Autodesk Inventor part; units mm, degrees
(part 2 of 5)
  circle A18 centre (0, 0) radius 45 construction
  circle A19 centre (0, 0) radius 45 construction
  line L916 (-38.7494, -0.2217) -> (-38.749, -0.2771)
  line L917 (-38.749, -0.2771) -> (-38.7743, -0.6234)
  line L918 (-38.7743, -0.6234) -> (-38.8288, -0.891)
  line L919 (-38.8288, -0.891) -> (-38.9042, -1.1194)
  line L920 (-38.9042, -1.1194) -> (-38.997, -1.3323)
  line L921 (-38.997, -1.3323) -> (-39.1059, -1.5242)
  line L922 (-39.1059, -1.5242) -> (-39.2291, -1.7067)
  line L923 (-39.2291, -1.7067) -> (-39.366, -1.8725)
  line L924 (-39.366, -1.8725) -> (-39.5158, -2.0289)
  line L925 (-39.5158, -2.0289) -> (-39.6781, -2.1727)
  line L926 (-39.6781, -2.1727) -> (-39.8523, -2.3033)
  line L927 (-39.8523, -2.3033) -> (-40.0379, -2.4272)
  line L928 (-40.0379, -2.4272) -> (-40.2348, -2.5371)
  line L929 (-40.2348, -2.5371) -> (-40.4428, -2.6351)
  line L930 (-40.4428, -2.6351) -> (-40.661, -2.7274)
  line L931 (-41.9049, 3.0266) -> (-42.1825, 3.0578)
  line L932 (-40.661, -2.7274) -> (-40.8898, -2.8078)
  line L933 (-40.8898, -2.8078) -> (-41.1289, -2.8764)
  line L934 (-41.1289, -2.8764) -> (-41.3781, -2.9334)
  line L935 (-41.3781, -2.9334) -> (-41.6367, -2.9845)
  line L936 (-41.9049, -3.0266) -> (-42.1825, -3.0578)
  line L937 (-41.6367, -2.9845) -> (-41.9049, -3.0266)
  line L938 (-40.4428, 2.6351) -> (-40.661, 2.7274)
  line L939 (-42.1825, -3.0578) -> (-42.555, -3.1194)
  line L940 (-42.555, -3.1194) -> (-42.9254, -3.2087)
  line L941 (-43.2942, -3.3167) -> (-43.6617, -3.4402)
  line L942 (-43.6617, -3.4402) -> (-44.0279, -3.5774)
  line L943 (-44.0279, -3.5774) -> (-44.3927, -3.7271)
  line L944 (-42.9254, -3.2087) -> (-43.2942, -3.3167)
  line L945 (-39.5158, 2.0289) -> (-39.6781, 2.1727)
  line L946 (-39.2291, 1.7067) -> (-39.366, 1.8725)
  line L947 (-39.366, 1.8725) -> (-39.5158, 2.0289)
  line L948 (-44.7563, -3.8884) -> (-45.1184, -4.0607)
  line L949 (-47.2601, -5.3011) -> (-47.6113, -5.5395)
  line L950 (-46.9072, -5.0713) -> (-47.2601, -5.3011)
  line L951 (-46.5526, -4.8504) -> (-46.9072, -5.0713)
  line L952 (-46.1963, -4.6386) -> (-46.5526, -4.8504)
  line L953 (-45.8385, -4.4362) -> (-46.1963, -4.6386)
  line L954 (-45.4792, -4.2434) -> (-45.8385, -4.4362)
  line L955 (-45.1184, -4.0607) -> (-45.4792, -4.2434)
  line L956 (-47.6113, -5.5395) -> (-47.9606, -5.7865)
  line L957 (-47.9606, -5.7865) -> (-48.308, -6.0419)
  line L958 (-48.308, -6.0419) -> (-48.6534, -6.3055)
  line L959 (-48.6534, -6.3055) -> (-48.9968, -6.5771)
  line L960 (-48.9968, -6.5771) -> (-49.338, -6.8568)
  line L961 (-49.338, -6.8568) -> (-49.2867, -7.2162)
  line L962 (-49.2867, -7.2162) -> (-49.2328, -7.5752)
  line L963 (-49.2328, -7.5752) -> (-49.1763, -7.9338)
  line L964 (-49.1763, -7.9338) -> (-49.1172, -8.292)
  line L965 (-49.1172, -8.292) -> (-49.0554, -8.6498)
  line L966 (-44.3927, -3.7271) -> (-44.7563, -3.8884)
  line L967 (-39.1059, 1.5242) -> (-39.2291, 1.7067)
  line L968 (-44.3927, 3.7271) -> (-44.7563, 3.8884)
  line L969 (-44.0279, 3.5774) -> (-44.3927, 3.7271)
  line L970 (-43.6617, 3.4402) -> (-44.0279, 3.5774)
  line L971 (-43.2942, 3.3167) -> (-43.6617, 3.4402)
  line L972 (-42.9254, 3.2087) -> (-43.2942, 3.3167)
  line L973 (-42.555, 3.1194) -> (-42.9254, 3.2087)
  line L974 (-44.7563, 3.8884) -> (-45.1184, 4.0607)
  line L975 (-45.1184, 4.0607) -> (-45.4792, 4.2434)
  line L976 (-47.6113, 5.5395) -> (-47.9606, 5.7865)
  line L977 (-47.2601, 5.3011) -> (-47.6113, 5.5395)
  line L978 (-46.9072, 5.0713) -> (-47.2601, 5.3011)
  line L979 (-46.5526, 4.8504) -> (-46.9072, 5.0713)
  line L980 (-46.1963, 4.6386) -> (-46.5526, 4.8504)
  line L981 (-45.8385, 4.4362) -> (-46.1963, 4.6386)
  line L982 (-45.4792, 4.2434) -> (-45.8385, 4.4362)
  line L983 (-47.9606, 5.7865) -> (-48.308, 6.0419)
  line L984 (-48.6534, 6.3055) -> (-48.9968, 6.5771)
  line L985 (-48.9968, 6.5771) -> (-49.338, 6.8568)
  line L986 (-49.338, 6.8568) -> (-49.2867, 7.2162)
  line L987 (-49.2867, 7.2162) -> (-49.2328, 7.5752)
  line L988 (-49.2328, 7.5752) -> (-49.1763, 7.9338)
  line L989 (-49.1763, 7.9338) -> (-49.1172, 8.292)
  line L990 (-49.1172, 8.292) -> (-49.0554, 8.6498)
  line L991 (-48.308, 6.0419) -> (-48.6534, 6.3055)
  line L992 (-38.997, 1.3323) -> (-39.1059, 1.5242)
  line L993 (-38.9042, 1.1194) -> (-38.997, 1.3323)
  line L994 (-38.8288, 0.891) -> (-38.9042, 1.1194)
  line L995 (-38.7743, 0.6234) -> (-38.8288, 0.891)
  line L996 (-38.749, 0.2771) -> (-38.7743, 0.6234)
  line L997 (-38.7494, 0.2217) -> (-38.749, 0.2771)
  line L998 (-38.7496, 0.1663) -> (-38.7494, 0.2217)
  line L999 (-38.7498, 0.1108) -> (-38.7496, 0.1663)
  line L1000 (-38.75, 0.0554) -> (-38.7498, 0.1108)
  line L1001 (-38.75, 0) -> (-38.75, 0.0554)
  line L1002 (-38.0283, -11.529) -> (-38.2367, -11.4659)
  line L1003 (-38.2367, -11.4659) -> (-38.4534, -11.4129)
  line L1004 (-38.4534, -11.4129) -> (-38.6761, -11.377)
  line L1005 (-38.6761, -11.377) -> (-38.905, -11.3561)
  line L1006 (-39.1417, -11.344) -> (-39.3842, -11.3467)
  line L1007 (-39.3842, -11.3467) -> (-39.6323, -11.364)
  line L1008 (-39.6323, -11.364) -> (-39.886, -11.3956)
  line L1009 (-39.886, -11.3956) -> (-40.1465, -11.4361)
  line L1010 (-40.1465, -11.4361) -> (-40.4129, -11.4882)
  line L1011 (-36.4131, -13.2533) -> (-36.3941, -13.3053)
  line L1012 (-36.3941, -13.3053) -> (-36.375, -13.3574)
  line L1013 (-36.375, -13.3574) -> (-36.3559, -13.4094)
  line L1014 (-36.3559, -13.4094) -> (-36.3367, -13.4614)
  line L1015 (-40.6845, -11.5538) -> (-41.0555, -11.6234)
  circle A20 centre (0, 0) radius 45 construction
  circle A21 centre (0, 0) radius 45 construction
  line L1016 (-36.3367, -13.4614) -> (-36.3174, -13.5133)
  line L1017 (-36.3174, -13.5133) -> (-36.2227, -13.8474)
  line L1018 (-36.2227, -13.8474) -> (-36.1824, -14.1175)
  line L1019 (-36.1824, -14.1175) -> (-36.1751, -14.3579)
  line L1020 (-36.1751, -14.3579) -> (-36.1896, -14.5898)
  line L1021 (-36.1896, -14.5898) -> (-36.2262, -14.8073)
  line L1022 (-36.2262, -14.8073) -> (-36.2795, -15.0209)
  line L1023 (-36.2795, -15.0209) -> (-36.3516, -15.2235)
  line L1024 (-36.3516, -15.2235) -> (-36.4388, -15.4218)
  line L1025 (-36.4388, -15.4218) -> (-36.5421, -15.6124)
  line L1026 (-36.5421, -15.6124) -> (-36.6611, -15.7947)
  line L1027 (-36.6611, -15.7947) -> (-36.7931, -15.9746)
  line L1028 (-36.7931, -15.9746) -> (-36.9406, -16.1452)
  line L1029 (-36.9406, -16.1452) -> (-37.1025, -16.3084)
  line L1030 (-37.1025, -16.3084) -> (-37.2761, -16.4698)
  line L1031 (-40.4129, -11.4882) -> (-40.6845, -11.5538)
  line L1032 (-37.2761, -16.4698) -> (-37.4636, -16.6236)
  line L1033 (-37.4636, -16.6236) -> (-37.6648, -16.7698)
  line L1034 (-37.6648, -16.7698) -> (-37.8794, -16.9086)
  line L1035 (-37.8794, -16.9086) -> (-38.105, -17.0451)
  line L1036 (-38.3425, -17.1764) -> (-38.5928, -17.3007)
  line L1037 (-38.105, -17.0451) -> (-38.3425, -17.1764)
  line L1038 (-38.905, -11.3561) -> (-39.1417, -11.344)
  line L1039 (-38.5928, -17.3007) -> (-38.9217, -17.4859)
  line L1040 (-38.9217, -17.4859) -> (-39.2392, -17.6965)
  line L1041 (-39.5489, -17.9241) -> (-39.852, -18.1659)
  line L1042 (-39.852, -18.1659) -> (-40.1491, -18.4201)
  line L1043 (-40.1491, -18.4201) -> (-40.4408, -18.6855)
  line L1044 (-39.2392, -17.6965) -> (-39.5489, -17.9241)
  line L1045 (-37.8267, -11.6087) -> (-38.0283, -11.529)
  line L1046 (-37.447, -11.8133) -> (-37.6324, -11.7044)
  line L1047 (-37.6324, -11.7044) -> (-37.8267, -11.6087)
  line L1048 (-40.7272, -18.9615) -> (-41.0086, -19.2472)
  line L1049 (-42.5969, -21.1453) -> (-42.8453, -21.4895)
  line L1050 (-42.3439, -20.8086) -> (-42.5969, -21.1453)
  line L1051 (-42.0862, -20.4798) -> (-42.3439, -20.8086)
  line L1052 (-41.8239, -20.1589) -> (-42.0862, -20.4798)
  line L1053 (-41.5569, -19.8464) -> (-41.8239, -20.1589)
  line L1054 (-41.2851, -19.5423) -> (-41.5569, -19.8464)
  line L1055 (-41.0086, -19.2472) -> (-41.2851, -19.5423)
  line L1056 (-42.8453, -21.4895) -> (-43.0891, -21.841)
  line L1057 (-43.0891, -21.841) -> (-43.3282, -22.1998)
  line L1058 (-43.3282, -22.1998) -> (-43.5626, -22.5656)
  line L1059 (-43.5626, -22.5656) -> (-43.7924, -22.9383)
  line L1060 (-43.7924, -22.9383) -> (-44.0174, -23.3178)
  line L1061 (-44.0174, -23.3178) -> (-43.8463, -23.638)
  line L1062 (-43.8463, -23.638) -> (-43.6728, -23.957)
  line L1063 (-43.6728, -23.957) -> (-43.4971, -24.2746)
  line L1064 (-43.4971, -24.2746) -> (-43.319, -24.591)
  line L1065 (-43.319, -24.591) -> (-43.1386, -24.9061)
  line L1066 (-40.4408, -18.6855) -> (-40.7272, -18.9615)
  line L1067 (-37.2688, -11.9427) -> (-37.447, -11.8133)
  line L1068 (-42.9903, -11.6809) -> (-43.387, -11.6536)
  line L1069 (-42.5962, -11.6968) -> (-42.9903, -11.6809)
  line L1070 (-42.2052, -11.7005) -> (-42.5962, -11.6968)
  line L1071 (-41.8176, -11.6908) -> (-42.2052, -11.7005)
  line L1072 (-41.4341, -11.6662) -> (-41.8176, -11.6908)
  line L1073 (-41.0555, -11.6234) -> (-41.4341, -11.6662)
  line L1074 (-43.387, -11.6536) -> (-43.7863, -11.6156)
  line L1075 (-43.7863, -11.6156) -> (-44.1878, -11.5673)
  line L1076 (-46.6346, -11.0786) -> (-47.0473, -10.9659)
  line L1077 (-46.223, -11.1825) -> (-46.6346, -11.0786)
  line L1078 (-45.8128, -11.2778) -> (-46.223, -11.1825)
  line L1079 (-45.4041, -11.3641) -> (-45.8128, -11.2778)
  line L1080 (-44.9969, -11.4412) -> (-45.4041, -11.3641)
  line L1081 (-44.5914, -11.509) -> (-44.9969, -11.4412)
  line L1082 (-44.1878, -11.5673) -> (-44.5914, -11.509)
  line L1083 (-47.0473, -10.9659) -> (-47.4611, -10.8448)
  line L1084 (-47.8758, -10.7152) -> (-48.2914, -10.5774)
  line L1085 (-48.2914, -10.5774) -> (-48.7077, -10.4313)
  line L1086 (-48.7077, -10.4313) -> (-48.7824, -10.0761)
  line L1087 (-48.7824, -10.0761) -> (-48.8546, -9.7203)
  line L1088 (-48.8546, -9.7203) -> (-48.9241, -9.3639)
  line L1089 (-48.9241, -9.3639) -> (-48.9911, -9.0071)
  line L1090 (-48.9911, -9.0071) -> (-49.0554, -8.6498)
  line L1091 (-47.4611, -10.8448) -> (-47.8758, -10.7152)
  line L1092 (-37.1009, -12.0858) -> (-37.2688, -11.9427)
  line L1093 (-36.9408, -12.2541) -> (-37.1009, -12.0858)
  line L1094 (-36.7919, -12.4429) -> (-36.9408, -12.2541)
  line L1095 (-36.6492, -12.6758) -> (-36.7919, -12.4429)
  line L1096 (-36.5069, -12.9926) -> (-36.6492, -12.6758)
  line L1097 (-36.4883, -13.0448) -> (-36.5069, -12.9926)
  line L1098 (-36.4696, -13.0969) -> (-36.4883, -13.0448)
  line L1099 (-36.4508, -13.1491) -> (-36.4696, -13.0969)
  line L1100 (-36.432, -13.2012) -> (-36.4508, -13.1491)
  line L1101 (-36.4131, -13.2533) -> (-36.432, -13.2012)
  line L1102 (-31.7918, -23.8401) -> (-32.0092, -23.8521)
  line L1103 (-32.0092, -23.8521) -> (-32.231, -23.8765)
  line L1104 (-32.231, -23.8765) -> (-32.4525, -23.9189)
  line L1105 (-32.4525, -23.9189) -> (-32.6748, -23.9775)
  line L1106 (-32.9013, -24.0471) -> (-33.1282, -24.1326)
  line L1107 (-33.1282, -24.1326) -> (-33.3555, -24.2337)
  line L1108 (-33.3555, -24.2337) -> (-33.583, -24.3502)
  line L1109 (-33.583, -24.3502) -> (-33.814, -24.4773)
  line L1110 (-33.814, -24.4773) -> (-34.0465, -24.6174)
  line L1111 (-29.6842, -24.908) -> (-29.6486, -24.9504)
  line L1112 (-29.6486, -24.9504) -> (-29.6129, -24.9928)
  line L1113 (-29.6129, -24.9928) -> (-29.5771, -25.0351)
  line L1114 (-29.5771, -25.0351) -> (-29.5412, -25.0774)
  line L1115 (-34.2792, -24.772) -> (-34.6041, -24.9642)
  circle A22 centre (0, 0) radius 45 construction
  circle A23 centre (0, 0) radius 45 construction
  line L1116 (-29.5412, -25.0774) -> (-29.5054, -25.1196)
  line L1117 (-29.5054, -25.1196) -> (-29.3021, -25.4012)
  line L1118 (-29.3021, -25.4012) -> (-29.1718, -25.6412)
  line L1119 (-29.1718, -25.6412) -> (-29.0828, -25.8646)
  line L1120 (-29.0828, -25.8646) -> (-29.0171, -26.0875)
  line L1121 (-29.0171, -26.0875) -> (-28.9771, -26.3044)
  line L1122 (-28.9771, -26.3044) -> (-28.9541, -26.5234)
  line L1123 (-28.9541, -26.5234) -> (-28.9525, -26.7384)
  line L1124 (-28.9525, -26.7384) -> (-28.9667, -26.9545)
  line L1125 (-28.9667, -26.9545) -> (-28.9985, -27.169)
  line L1126 (-28.9985, -27.169) -> (-29.0481, -27.381)
  line L1127 (-29.0481, -27.381) -> (-29.1106, -27.5952)
  line L1128 (-29.1106, -27.5952) -> (-29.1908, -27.806)
  line L1129 (-29.1908, -27.806) -> (-29.2872, -28.0147)
  line L1130 (-29.2872, -28.0147) -> (-29.395, -28.2257)
  line L1131 (-34.0465, -24.6174) -> (-34.2792, -24.772)
  line L1132 (-29.395, -28.2257) -> (-29.5186, -28.4343)
  line L1133 (-29.5186, -28.4343) -> (-29.6577, -28.6406)
  line L1134 (-29.6577, -28.6406) -> (-29.8119, -28.8444)
  line L1135 (-29.8119, -28.8444) -> (-29.9772, -29.0498)
  line L1136 (-30.1555, -29.2545) -> (-30.3482, -29.4569)
  line L1137 (-29.9772, -29.0498) -> (-30.1555, -29.2545)
  line L1138 (-32.6748, -23.9775) -> (-32.9013, -24.0471)
  line L1139 (-30.3482, -29.4569) -> (-30.5939, -29.7434)
  line L1140 (-30.5939, -29.7434) -> (-30.8202, -30.0499)
  line L1141 (-31.0334, -30.3697) -> (-31.2355, -30.7005)
  line L1142 (-31.2355, -30.7005) -> (-31.4278, -31.041)
  line L1143 (-31.4278, -31.041) -> (-31.6111, -31.3902)
  line L1144 (-30.8202, -30.0499) -> (-31.0334, -30.3697)
  line L1145 (-31.575, -23.8461) -> (-31.7918, -23.8401)
  line L1146 (-31.1483, -23.9085) -> (-31.3597, -23.8696)
  line L1147 (-31.3597, -23.8696) -> (-31.575, -23.8461)
  line L1148 (-31.7858, -31.7475) -> (-31.9525, -32.1123)
  line L1149 (-32.7959, -34.4391) -> (-32.9116, -34.8475)
  line L1150 (-32.6732, -34.0362) -> (-32.7959, -34.4391)
  line L1151 (-32.5436, -33.639) -> (-32.6732, -34.0362)
  line L1152 (-32.4068, -33.2478) -> (-32.5436, -33.639)
  line L1153 (-32.2628, -32.8628) -> (-32.4068, -33.2478)
  line L1154 (-32.1115, -32.4841) -> (-32.2628, -32.8628)
  line L1155 (-31.9525, -32.1123) -> (-32.1115, -32.4841)
  line L1156 (-32.9116, -34.8475) -> (-33.0204, -35.2612)
  line L1157 (-33.0204, -35.2612) -> (-33.1224, -35.6801)
  line L1158 (-33.1224, -35.6801) -> (-33.2176, -36.1041)
  line L1159 (-33.2176, -36.1041) -> (-33.306, -36.5329)
  line L1160 (-33.306, -36.5329) -> (-33.3877, -36.9664)
  line L1161 (-33.3877, -36.9664) -> (-33.1173, -37.2088)
  line L1162 (-33.1173, -37.2088) -> (-32.8453, -37.4492)
  line L1163 (-32.8453, -37.4492) -> (-32.5715, -37.6876)
  line L1164 (-32.5715, -37.6876) -> (-32.2959, -37.924)
  line L1165 (-32.2959, -37.924) -> (-32.0186, -38.1583)
  line L1166 (-31.6111, -31.3902) -> (-31.7858, -31.7475)
  line L1167 (-30.9366, -23.9692) -> (-31.1483, -23.9085)
  line L1168 (-36.4025, -25.68) -> (-36.7847, -25.7901)
  line L1169 (-36.0268, -25.5601) -> (-36.4025, -25.68)
  line L1170 (-35.6581, -25.4299) -> (-36.0268, -25.5601)
  line L1171 (-35.2972, -25.2883) -> (-35.6581, -25.4299)
  line L1172 (-34.9452, -25.1339) -> (-35.2972, -25.2883)
  line L1173 (-34.6041, -24.9642) -> (-34.9452, -25.1339)
  line L1174 (-36.7847, -25.7901) -> (-37.1729, -25.8909)
  line L1175 (-37.1729, -25.8909) -> (-37.5667, -25.9828)
  line L1176 (-40.0331, -26.3604) -> (-40.4594, -26.3957)
  line L1177 (-39.6108, -26.3174) -> (-40.0331, -26.3604)
  line L1178 (-39.1928, -26.2665) -> (-39.6108, -26.3174)
  line L1179 (-38.7791, -26.2078) -> (-39.1928, -26.2665)
  line L1180 (-38.3701, -26.1411) -> (-38.7791, -26.2078)
  line L1181 (-37.9659, -26.0661) -> (-38.3701, -26.1411)
  line L1182 (-37.5667, -25.9828) -> (-37.9659, -26.0661)
  line L1183 (-40.4594, -26.3957) -> (-40.8897, -26.4234)
  line L1184 (-41.3237, -26.4435) -> (-41.7614, -26.4561)
  line L1185 (-41.7614, -26.4561) -> (-42.2025, -26.4613)
  line L1186 (-42.2025, -26.4613) -> (-42.3943, -26.153)
  line L1187 (-42.3943, -26.153) -> (-42.5838, -25.8433)
  line L1188 (-42.5838, -25.8433) -> (-42.771, -25.5322)
  line L1189 (-42.771, -25.5322) -> (-42.9559, -25.2198)
  line L1190 (-42.9559, -25.2198) -> (-43.1386, -24.9061)
  line L1191 (-40.8897, -26.4234) -> (-41.3237, -26.4435)
  line L1192 (-30.7299, -24.0462) -> (-30.9366, -23.9692)
  line L1193 (-30.5219, -24.1496) -> (-30.7299, -24.0462)
  line L1194 (-30.3173, -24.2761) -> (-30.5219, -24.1496)
  line L1195 (-30.1036, -24.4461) -> (-30.3173, -24.2761)
  line L1196 (-29.8616, -24.6951) -> (-30.1036, -24.4461)
  line L1197 (-29.8262, -24.7378) -> (-29.8616, -24.6951)
  line L1198 (-29.7908, -24.7804) -> (-29.8262, -24.7378)
  line L1199 (-29.7553, -24.823) -> (-29.7908, -24.7804)
  line L1200 (-29.7198, -24.8655) -> (-29.7553, -24.823)
  line L1201 (-29.6842, -24.908) -> (-29.7198, -24.8655)
  line L1202 (-21.7207, -33.2758) -> (-21.9209, -33.3615)
  line L1203 (-21.9209, -33.3615) -> (-22.121, -33.4602)
  line L1204 (-22.121, -33.4602) -> (-22.3146, -33.5758)
  line L1205 (-22.3146, -33.5758) -> (-22.5034, -33.7069)
  line L1206 (-22.6925, -33.8498) -> (-22.8765, -34.0078)
  line L1207 (-22.8765, -34.0078) -> (-23.0555, -34.1805)
  line L1208 (-23.0555, -34.1805) -> (-23.2294, -34.3678)
  line L1209 (-23.2294, -34.3678) -> (-23.403, -34.5662)
  line L1210 (-23.403, -34.5662) -> (-23.5736, -34.7774)
  line L1211 (-19.375, -33.5585) -> (-19.327, -33.5862)
  line L1212 (-19.327, -33.5862) -> (-19.2789, -33.6138)
  line L1213 (-19.2789, -33.6138) -> (-19.2308, -33.6413)
  line L1214 (-19.2308, -33.6413) -> (-19.1827, -33.6688)
  line L1215 (-23.7394, -35.0022) -> (-23.979, -35.294)
  circle A24 centre (0, 0) radius 45 construction
  circle A25 centre (0, 0) radius 45 construction
  line L1216 (-19.1827, -33.6688) -> (-19.1345, -33.6962)
  line L1217 (-19.1345, -33.6962) -> (-18.8473, -33.8913)
  line L1218 (-18.8473, -33.8913) -> (-18.6427, -34.0722)
  line L1219 (-18.6427, -34.0722) -> (-18.4826, -34.2517)
  line L1220 (-18.4826, -34.2517) -> (-18.3447, -34.4386)
  line L1221 (-18.3447, -34.4386) -> (-18.2329, -34.6288)
  line L1222 (-18.2329, -34.6288) -> (-18.1365, -34.8267)
  line L1223 (-18.1365, -34.8267) -> (-18.0614, -35.0282)
  line L1224 (-18.0614, -35.0282) -> (-18.0008, -35.2362)
  line L1225 (-18.0008, -35.2362) -> (-17.9574, -35.4486)
  line L1226 (-17.9574, -35.4486) -> (-17.9314, -35.6648)
  line L1227 (-17.9314, -35.6648) -> (-17.9169, -35.8874)
  line L1228 (-17.9169, -35.8874) -> (-17.9202, -36.1129)
  line L1229 (-17.9202, -36.1129) -> (-17.9393, -36.342)
  line L1230 (-17.9393, -36.342) -> (-17.9685, -36.5772)
  line L1231 (-23.5736, -34.7774) -> (-23.7394, -35.0022)
  line L1232 (-17.9685, -36.5772) -> (-18.0133, -36.8155)
  line L1233 (-18.0133, -36.8155) -> (-18.0734, -37.0569)
  line L1234 (-18.0734, -37.0569) -> (-18.1486, -37.3012)
  line L1235 (-18.1486, -37.3012) -> (-18.2337, -37.5507)
  line L1236 (-18.3313, -37.804) -> (-18.4431, -38.0601)
  line L1237 (-18.2337, -37.5507) -> (-18.3313, -37.804)
  line L1238 (-22.5034, -33.7069) -> (-22.6925, -33.8498)
  line L1239 (-18.4431, -38.0601) -> (-18.576, -38.4134)
  line L1240 (-18.576, -38.4134) -> (-18.6839, -38.7788)
  line L1241 (-18.7748, -39.1522) -> (-18.8516, -39.5322)
  line L1242 (-18.8516, -39.5322) -> (-18.9158, -39.9179)
  line L1243 (-18.9158, -39.9179) -> (-18.9686, -40.3088)
  line L1244 (-18.6839, -38.7788) -> (-18.7748, -39.1522)
  line L1245 (-21.515, -33.2073) -> (-21.7207, -33.2758)
  line L1246 (-21.0926, -33.12) -> (-21.3046, -33.1558)
  line L1247 (-21.3046, -33.1558) -> (-21.515, -33.2073)
  line L1248 (-19.0107, -40.7043) -> (-19.0425, -41.1041)
  line L1249 (-19.0392, -43.579) -> (-19.0083, -44.0023)
  line L1250 (-19.0617, -43.1585) -> (-19.0392, -43.579)
  line L1251 (-19.0757, -42.7409) -> (-19.0617, -43.1585)
  line L1252 (-19.081, -42.3265) -> (-19.0757, -42.7409)
  line L1253 (-19.0774, -41.9154) -> (-19.081, -42.3265)
  line L1254 (-19.0647, -41.5079) -> (-19.0774, -41.9154)
  line L1255 (-19.0425, -41.1041) -> (-19.0647, -41.5079)
  line L1256 (-19.0083, -44.0023) -> (-18.969, -44.4283)
  line L1257 (-18.969, -44.4283) -> (-18.9216, -44.8569)
  line L1258 (-18.9216, -44.8569) -> (-18.866, -45.2878)
  line L1259 (-18.866, -45.2878) -> (-18.8024, -45.721)
  line L1260 (-18.8024, -45.721) -> (-18.7309, -46.1563)
  line L1261 (-18.7309, -46.1563) -> (-18.394, -46.2916)
  line L1262 (-18.394, -46.2916) -> (-18.0561, -46.4245)
  line L1263 (-18.0561, -46.4245) -> (-17.7172, -46.5548)
  line L1264 (-17.7172, -46.5548) -> (-17.3775, -46.6827)
  line L1265 (-17.3775, -46.6827) -> (-17.0368, -46.8081)
  line L1266 (-18.9686, -40.3088) -> (-19.0107, -40.7043)
  line L1267 (-20.8729, -33.1046) -> (-21.0926, -33.12)
  line L1268 (-25.4241, -36.5817) -> (-25.7456, -36.8158)
  line L1269 (-25.1121, -36.3405) -> (-25.4241, -36.5817)
  line L1270 (-24.8101, -36.092) -> (-25.1121, -36.3405)
  line L1271 (-24.5194, -35.8356) -> (-24.8101, -36.092)
  line L1272 (-24.2415, -35.5701) -> (-24.5194, -35.8356)
  line L1273 (-23.979, -35.294) -> (-24.2415, -35.5701)
  line L1274 (-25.7456, -36.8158) -> (-26.0759, -37.0434)
  line L1275 (-26.0759, -37.0434) -> (-26.4145, -37.2644)
  line L1276 (-28.603, -38.4628) -> (-28.9916, -38.6418)
  line L1277 (-28.2209, -38.2779) -> (-28.603, -38.4628)
  line L1278 (-27.8455, -38.0872) -> (-28.2209, -38.2779)
  line L1279 (-27.4768, -37.8905) -> (-27.8455, -38.0872)
  line L1280 (-27.1153, -37.6879) -> (-27.4768, -37.8905)
  line L1281 (-26.7611, -37.4792) -> (-27.1153, -37.6879)
  line L1282 (-26.4145, -37.2644) -> (-26.7611, -37.4792)
  line L1283 (-28.9916, -38.6418) -> (-29.3864, -38.815)
  line L1284 (-29.7874, -38.9823) -> (-30.1943, -39.1439)
  line L1285 (-30.1943, -39.1439) -> (-30.6071, -39.2996)
  line L1286 (-30.6071, -39.2996) -> (-30.8927, -39.0755)
  line L1287 (-30.8927, -39.0755) -> (-31.1767, -38.8493)
  line L1288 (-31.1767, -38.8493) -> (-31.459, -38.621)
  line L1289 (-31.459, -38.621) -> (-31.7397, -38.3907)
  line L1290 (-31.7397, -38.3907) -> (-32.0186, -38.1583)
  line L1291 (-29.3864, -38.815) -> (-29.7874, -38.9823)
  line L1292 (-20.6524, -33.1063) -> (-20.8729, -33.1046)
  line L1293 (-20.4215, -33.1323) -> (-20.6524, -33.1063)
  line L1294 (-20.186, -33.1812) -> (-20.4215, -33.1323)
  line L1295 (-19.9271, -33.2679) -> (-20.186, -33.1812)
  line L1296 (-19.6145, -33.4191) -> (-19.9271, -33.2679)
  line L1297 (-19.5667, -33.4471) -> (-19.6145, -33.4191)
  line L1298 (-19.5188, -33.475) -> (-19.5667, -33.4471)
  line L1299 (-19.4709, -33.5029) -> (-19.5188, -33.475)
  line L1300 (-19.423, -33.5307) -> (-19.4709, -33.5029)
  line L1301 (-19.375, -33.5585) -> (-19.423, -33.5307)
  line L1302 (-9.0298, -38.698) -> (-9.1886, -38.8469)
  line L1303 (-9.1886, -38.8469) -> (-9.3428, -39.0081)
  line L1304 (-9.3428, -39.0081) -> (-9.4853, -39.183)
  line L1305 (-9.4853, -39.183) -> (-9.6179, -39.3708)
  line L1306 (-9.7467, -39.5697) -> (-9.8655, -39.7811)
  line L1307 (-9.8655, -39.7811) -> (-9.9747, -40.0046)
  line L1308 (-9.9747, -40.0046) -> (-10.0741, -40.2401)
  line L1309 (-10.0741, -40.2401) -> (-10.1693, -40.4859)
  line L1310 (-10.1693, -40.4859) -> (-10.2574, -40.7427)
  line L1311 (-6.7289, -38.1613) -> (-6.6743, -38.1709)
  line L1312 (-6.6743, -38.1709) -> (-6.6197, -38.1804)
  line L1313 (-6.6197, -38.1804) -> (-6.5651, -38.1898)
  line L1314 (-6.5651, -38.1898) -> (-6.5105, -38.1992)
  line L1315 (-10.3363, -41.0107) -> (-10.4616, -41.3668)
  circle A26 centre (0, 0) radius 45 construction
  circle A27 centre (0, 0) radius 45 construction
  line L1316 (-6.5105, -38.1992) -> (-6.4558, -38.2084)
  line L1317 (-6.4558, -38.2084) -> (-6.1191, -38.2935)
  line L1318 (-6.1191, -38.2935) -> (-5.8651, -38.3936)
  line L1319 (-5.8651, -38.3936) -> (-5.6532, -38.5075)
  line L1320 (-5.6532, -38.5075) -> (-5.4597, -38.636)
  line L1321 (-5.4597, -38.636) -> (-5.2896, -38.7764)
  line L1322 (-5.2896, -38.7764) -> (-5.1313, -38.9295)
  line L1323 (-5.1313, -38.9295) -> (-4.9918, -39.0931)
  line L1324 (-4.9918, -39.0931) -> (-4.8638, -39.2678)
  line L1325 (-4.8638, -39.2678) -> (-4.7503, -39.4526)
  line L1326 (-4.7503, -39.4526) -> (-4.6519, -39.6468)
  line L1327 (-4.6519, -39.6468) -> (-4.5622, -39.8511)
  line L1328 (-4.5622, -39.8511) -> (-4.4881, -40.0641)
  line L1329 (-4.4881, -40.0641) -> (-4.4278, -40.2859)
  line L1330 (-4.4278, -40.2859) -> (-4.3747, -40.5169)
  line L1331 (-10.2574, -40.7427) -> (-10.3363, -41.0107)
  line L1332 (-4.3747, -40.5169) -> (-4.3353, -40.7562)
  line L1333 (-4.3353, -40.7562) -> (-4.3093, -41.0036)
  line L1334 (-4.3093, -41.0036) -> (-4.2964, -41.2588)
  line L1335 (-4.2964, -41.2588) -> (-4.291, -41.5224)
  line L1336 (-4.2961, -41.7938) -> (-4.3135, -42.0727)
  line L1337 (-4.291, -41.5224) -> (-4.2961, -41.7938)
  line L1338 (-9.6179, -39.3708) -> (-9.7467, -39.5697)
  line L1339 (-4.3135, -42.0727) -> (-4.3176, -42.4502)
  line L1340 (-4.3176, -42.4502) -> (-4.294, -42.8304)
  line L1341 (-4.2517, -43.2124) -> (-4.1939, -43.5958)
  line L1342 (-4.1939, -43.5958) -> (-4.1223, -43.9802)
  line L1343 (-4.1223, -43.9802) -> (-4.0382, -44.3655)
  line L1344 (-4.294, -42.8304) -> (-4.2517, -43.2124)
  line L1345 (-8.8599, -38.5632) -> (-9.0298, -38.698)
  line L1346 (-8.4928, -38.3367) -> (-8.6799, -38.4428)
  line L1347 (-8.6799, -38.4428) -> (-8.8599, -38.5632)
  line L1348 (-3.9425, -44.7515) -> (-3.8357, -45.1381)
  line L1349 (-2.9861, -47.4626) -> (-2.8122, -47.8499)
  line L1350 (-3.1511, -47.0752) -> (-2.9861, -47.4626)
  line L1351 (-3.3071, -46.6876) -> (-3.1511, -47.0752)
  line L1352 (-3.4538, -46.3) -> (-3.3071, -46.6876)
  line L1353 (-3.591, -45.9125) -> (-3.4538, -46.3)
  line L1354 (-3.7184, -45.5251) -> (-3.591, -45.9125)
  line L1355 (-3.8357, -45.1381) -> (-3.7184, -45.5251)
  line L1356 (-2.8122, -47.8499) -> (-2.6297, -48.2368)
  line L1357 (-2.6297, -48.2368) -> (-2.4385, -48.6232)
  line L1358 (-2.4385, -48.6232) -> (-2.2389, -49.0092)
  line L1359 (-2.2389, -49.0092) -> (-2.031, -49.3945)
  line L1360 (-2.031, -49.3945) -> (-1.8149, -49.7791)
  line L1361 (-1.8149, -49.7791) -> (-1.452, -49.791)
  line L1362 (-1.452, -49.791) -> (-1.0891, -49.8003)
  line L1363 (-1.0891, -49.8003) -> (-0.7261, -49.8069)
  line L1364 (-0.7261, -49.8069) -> (-0.363, -49.8108)
  line L1365 (-0.363, -49.8108) -> (0, -49.8122)
  line L1366 (-4.0382, -44.3655) -> (-3.9425, -44.7515)
  line L1367 (-8.2917, -38.2471) -> (-8.4928, -38.3367)
  line L1368 (-11.3792, -43.0711) -> (-11.6012, -43.4011)
  line L1369 (-11.1684, -42.7378) -> (-11.3792, -43.0711)
  line L1370 (-10.9697, -42.401) -> (-11.1684, -42.7378)
  line L1371 (-10.7842, -42.0605) -> (-10.9697, -42.401)
  line L1372 (-10.6138, -41.716) -> (-10.7842, -42.0605)
  line L1373 (-10.4616, -41.3668) -> (-10.6138, -41.716)
  line L1374 (-11.6012, -43.4011) -> (-11.8338, -43.7278)
  line L1375 (-11.8338, -43.7278) -> (-12.0764, -44.0514)
  line L1376 (-13.723, -45.926) -> (-14.0269, -46.2271)
  line L1377 (-13.4272, -45.6216) -> (-13.723, -45.926)
  line L1378 (-13.1396, -45.314) -> (-13.4272, -45.6216)
  line L1379 (-12.8605, -45.0031) -> (-13.1396, -45.314)
  line L1380 (-12.59, -44.689) -> (-12.8605, -45.0031)
  line L1381 (-12.3286, -44.3718) -> (-12.59, -44.689)
  line L1382 (-12.0764, -44.0514) -> (-12.3286, -44.3718)
  line L1383 (-14.0269, -46.2271) -> (-14.3387, -46.5249)
  line L1384 (-14.6582, -46.8193) -> (-14.9854, -47.1103)
  line L1385 (-14.9854, -47.1103) -> (-15.32, -47.3978)
  line L1386 (-15.32, -47.3978) -> (-15.6651, -47.2849)
  line L1387 (-15.6651, -47.2849) -> (-16.0093, -47.1694)
  line L1388 (-16.0093, -47.1694) -> (-16.3527, -47.0515)
  line L1389 (-16.3527, -47.0515) -> (-16.6952, -46.9311)
  line L1390 (-16.6952, -46.9311) -> (-17.0368, -46.8081)
  line L1391 (-14.3387, -46.5249) -> (-14.6582, -46.8193)
  line L1392 (-8.0839, -38.1732) -> (-8.2917, -38.2471)
  line L1393 (-7.8581, -38.1187) -> (-8.0839, -38.1732)
  line L1394 (-7.62, -38.0842) -> (-7.8581, -38.1187)
  line L1395 (-7.347, -38.077) -> (-7.62, -38.0842)
  line L1396 (-7.0016, -38.1122) -> (-7.347, -38.077)
  line L1397 (-6.9471, -38.1222) -> (-7.0016, -38.1122)
  line L1398 (-6.8925, -38.1321) -> (-6.9471, -38.1222)
  line L1399 (-6.838, -38.1419) -> (-6.8925, -38.1321)
  line L1400 (-6.7834, -38.1516) -> (-6.838, -38.1419)
  line L1401 (-6.7289, -38.1613) -> (-6.7834, -38.1516)
  line L1402 (4.7503, -39.4526) -> (4.6519, -39.6468)
  line L1403 (4.6519, -39.6468) -> (4.5622, -39.8511)
  line L1404 (4.5622, -39.8511) -> (4.4881, -40.0641)
  line L1405 (4.4881, -40.0641) -> (4.4278, -40.2859)
  line L1406 (4.3747, -40.5169) -> (4.3353, -40.7562)
  line L1407 (4.3353, -40.7562) -> (4.3093, -41.0036)
  line L1408 (4.3093, -41.0036) -> (4.2964, -41.2588)
  line L1409 (4.2964, -41.2588) -> (4.291, -41.5224)
  line L1410 (4.291, -41.5224) -> (4.2961, -41.7938)
  line L1411 (6.7289, -38.1613) -> (6.7834, -38.1516)
  line L1412 (6.7834, -38.1516) -> (6.838, -38.1419)
  line L1413 (6.838, -38.1419) -> (6.8925, -38.1321)
  line L1414 (6.8925, -38.1321) -> (6.9471, -38.1222)
  line L1415 (4.3135, -42.0727) -> (4.3176, -42.4502)
  circle A28 centre (0, 0) radius 45 construction
  circle A29 centre (0, 0) radius 45 construction
  line L1416 (6.9471, -38.1222) -> (7.0016, -38.1122)
  line L1417 (7.0016, -38.1122) -> (7.347, -38.077)
  line L1418 (7.347, -38.077) -> (7.62, -38.0842)
  line L1419 (7.62, -38.0842) -> (7.8581, -38.1187)
  line L1420 (7.8581, -38.1187) -> (8.0839, -38.1732)
  line L1421 (8.0839, -38.1732) -> (8.2917, -38.2471)
  line L1422 (8.2917, -38.2471) -> (8.4928, -38.3367)
  line L1423 (8.4928, -38.3367) -> (8.6799, -38.4428)
  line L1424 (8.6799, -38.4428) -> (8.8599, -38.5632)
  line L1425 (8.8599, -38.5632) -> (9.0298, -38.698)
  line L1426 (9.0298, -38.698) -> (9.1886, -38.8469)
  line L1427 (9.1886, -38.8469) -> (9.3428, -39.0081)
  line L1428 (9.3428, -39.0081) -> (9.4853, -39.183)
  line L1429 (9.4853, -39.183) -> (9.6179, -39.3708)
  line L1430 (9.6179, -39.3708) -> (9.7467, -39.5697)
  line L1431 (4.2961, -41.7938) -> (4.3135, -42.0727)
  line L1432 (9.7467, -39.5697) -> (9.8655, -39.7811)
  line L1433 (9.8655, -39.7811) -> (9.9747, -40.0046)
  line L1434 (9.9747, -40.0046) -> (10.0741, -40.2401)
  line L1435 (10.0741, -40.2401) -> (10.1693, -40.4859)
  line L1436 (10.2574, -40.7427) -> (10.3363, -41.0107)
  line L1437 (10.1693, -40.4859) -> (10.2574, -40.7427)
  line L1438 (4.4278, -40.2859) -> (4.3747, -40.5169)
  line L1439 (10.3363, -41.0107) -> (10.4616, -41.3668)
  line L1440 (10.4616, -41.3668) -> (10.6138, -41.716)
  line L1441 (10.7842, -42.0605) -> (10.9697, -42.401)
  line L1442 (10.9697, -42.401) -> (11.1684, -42.7378)
  line L1443 (11.1684, -42.7378) -> (11.3792, -43.0711)
  line L1444 (10.6138, -41.716) -> (10.7842, -42.0605)
  line L1445 (4.8638, -39.2678) -> (4.7503, -39.4526)
  line L1446 (5.1313, -38.9295) -> (4.9918, -39.0931)
  line L1447 (4.9918, -39.0931) -> (4.8638, -39.2678)
  line L1448 (11.6012, -43.4011) -> (11.8338, -43.7278)
  line L1449 (13.4272, -45.6216) -> (13.723, -45.926)
  line L1450 (13.1396, -45.314) -> (13.4272, -45.6216)
  line L1451 (12.8605, -45.0031) -> (13.1396, -45.314)
  line L1452 (12.59, -44.689) -> (12.8605, -45.0031)
  line L1453 (12.3286, -44.3718) -> (12.59, -44.689)
  line L1454 (12.0764, -44.0514) -> (12.3286, -44.3718)
  line L1455 (11.8338, -43.7278) -> (12.0764, -44.0514)
  line L1456 (13.723, -45.926) -> (14.0269, -46.2271)
  line L1457 (14.0269, -46.2271) -> (14.3387, -46.5249)
  line L1458 (14.3387, -46.5249) -> (14.6582, -46.8193)
  line L1459 (14.6582, -46.8193) -> (14.9854, -47.1103)
  line L1460 (14.9854, -47.1103) -> (15.32, -47.3978)
  line L1461 (15.32, -47.3978) -> (15.6651, -47.2849)
  line L1462 (15.6651, -47.2849) -> (16.0093, -47.1694)
  line L1463 (16.0093, -47.1694) -> (16.3527, -47.0515)
  line L1464 (16.3527, -47.0515) -> (16.6952, -46.9311)
  line L1465 (16.6952, -46.9311) -> (17.0368, -46.8081)
  line L1466 (11.3792, -43.0711) -> (11.6012, -43.4011)
  line L1467 (5.2896, -38.7764) -> (5.1313, -38.9295)
  line L1468 (4.0382, -44.3655) -> (3.9425, -44.7515)
  line L1469 (4.1223, -43.9802) -> (4.0382, -44.3655)
  line L1470 (4.1939, -43.5958) -> (4.1223, -43.9802)
  line L1471 (4.2517, -43.2124) -> (4.1939, -43.5958)
  line L1472 (4.294, -42.8304) -> (4.2517, -43.2124)
  line L1473 (4.3176, -42.4502) -> (4.294, -42.8304)
  line L1474 (3.9425, -44.7515) -> (3.8357, -45.1381)
  line L1475 (3.8357, -45.1381) -> (3.7184, -45.5251)
  line L1476 (2.8122, -47.8499) -> (2.6297, -48.2368)
  line L1477 (2.9861, -47.4626) -> (2.8122, -47.8499)
  line L1478 (3.1511, -47.0752) -> (2.9861, -47.4626)
  line L1479 (3.3071, -46.6876) -> (3.1511, -47.0752)
  line L1480 (3.4538, -46.3) -> (3.3071, -46.6876)
  line L1481 (3.591, -45.9125) -> (3.4538, -46.3)
  line L1482 (3.7184, -45.5251) -> (3.591, -45.9125)
  line L1483 (2.6297, -48.2368) -> (2.4385, -48.6232)
  line L1484 (2.2389, -49.0092) -> (2.031, -49.3945)
  line L1485 (2.031, -49.3945) -> (1.8149, -49.7791)
  line L1486 (1.8149, -49.7791) -> (1.452, -49.791)
  line L1487 (1.452, -49.791) -> (1.0891, -49.8003)
  line L1488 (1.0891, -49.8003) -> (0.7261, -49.8069)
  line L1489 (0.7261, -49.8069) -> (0.363, -49.8108)
  line L1490 (0.363, -49.8108) -> (0, -49.8122)
  line L1491 (2.4385, -48.6232) -> (2.2389, -49.0092)
  line L1492 (5.4597, -38.636) -> (5.2896, -38.7764)
  line L1493 (5.6532, -38.5075) -> (5.4597, -38.636)
  line L1494 (5.8651, -38.3936) -> (5.6532, -38.5075)
  line L1495 (6.1191, -38.2935) -> (5.8651, -38.3936)
  line L1496 (6.4558, -38.2084) -> (6.1191, -38.2935)
  line L1497 (6.5105, -38.1992) -> (6.4558, -38.2084)
  line L1498 (6.5651, -38.1898) -> (6.5105, -38.1992)
  line L1499 (6.6197, -38.1804) -> (6.5651, -38.1898)
  line L1500 (6.6743, -38.1709) -> (6.6197, -38.1804)
  line L1501 (6.7289, -38.1613) -> (6.6743, -38.1709)
  line L1502 (17.9574, -35.4486) -> (17.9314, -35.6648)
  line L1503 (17.9314, -35.6648) -> (17.9169, -35.8874)
  line L1504 (17.9169, -35.8874) -> (17.9202, -36.1129)
  line L1505 (17.9202, -36.1129) -> (17.9393, -36.342)
  line L1506 (17.9685, -36.5772) -> (18.0133, -36.8155)
  line L1507 (18.0133, -36.8155) -> (18.0734, -37.0569)
  line L1508 (18.0734, -37.0569) -> (18.1486, -37.3012)
  line L1509 (18.1486, -37.3012) -> (18.2337, -37.5507)
  line L1510 (18.2337, -37.5507) -> (18.3313, -37.804)
  line L1511 (19.375, -33.5585) -> (19.423, -33.5307)
  line L1512 (19.423, -33.5307) -> (19.4709, -33.5029)
  line L1513 (19.4709, -33.5029) -> (19.5188, -33.475)
  line L1514 (19.5188, -33.475) -> (19.5667, -33.4471)
  line L1515 (18.4431, -38.0601) -> (18.576, -38.4134)
  circle A30 centre (0, 0) radius 45 construction
  circle A31 centre (0, 0) radius 45 construction
  line L1516 (19.5667, -33.4471) -> (19.6145, -33.4191)
  line L1517 (19.6145, -33.4191) -> (19.9271, -33.2679)
  line L1518 (19.9271, -33.2679) -> (20.186, -33.1812)
  line L1519 (20.186, -33.1812) -> (20.4215, -33.1323)
  line L1520 (20.4215, -33.1323) -> (20.6524, -33.1063)
  line L1521 (20.6524, -33.1063) -> (20.8729, -33.1046)
  line L1522 (20.8729, -33.1046) -> (21.0926, -33.12)
  line L1523 (21.0926, -33.12) -> (21.3046, -33.1558)
  line L1524 (21.3046, -33.1558) -> (21.515, -33.2073)
  line L1525 (21.515, -33.2073) -> (21.7207, -33.2758)
  line L1526 (21.7207, -33.2758) -> (21.9209, -33.3615)
  line L1527 (21.9209, -33.3615) -> (22.121, -33.4602)
  line L1528 (22.121, -33.4602) -> (22.3146, -33.5758)
  line L1529 (22.3146, -33.5758) -> (22.5034, -33.7069)
  line L1530 (22.5034, -33.7069) -> (22.6925, -33.8498)
  line L1531 (18.3313, -37.804) -> (18.4431, -38.0601)
  line L1532 (22.6925, -33.8498) -> (22.8765, -34.0078)
  line L1533 (22.8765, -34.0078) -> (23.0555, -34.1805)
  line L1534 (23.0555, -34.1805) -> (23.2294, -34.3678)
  line L1535 (23.2294, -34.3678) -> (23.403, -34.5662)
  line L1536 (23.5736, -34.7774) -> (23.7394, -35.0022)
  line L1537 (23.403, -34.5662) -> (23.5736, -34.7774)
  line L1538 (17.9393, -36.342) -> (17.9685, -36.5772)
  line L1539 (23.7394, -35.0022) -> (23.979, -35.294)
  line L1540 (23.979, -35.294) -> (24.2415, -35.5701)
  line L1541 (24.5194, -35.8356) -> (24.8101, -36.092)
  line L1542 (24.8101, -36.092) -> (25.1121, -36.3405)
  line L1543 (25.1121, -36.3405) -> (25.4241, -36.5817)
  line L1544 (24.2415, -35.5701) -> (24.5194, -35.8356)
  line L1545 (18.0008, -35.2362) -> (17.9574, -35.4486)
  line L1546 (18.1365, -34.8267) -> (18.0614, -35.0282)
  line L1547 (18.0614, -35.0282) -> (18.0008, -35.2362)
  line L1548 (25.7456, -36.8158) -> (26.0759, -37.0434)
  line L1549 (28.2209, -38.2779) -> (28.603, -38.4628)
  line L1550 (27.8455, -38.0872) -> (28.2209, -38.2779)
  line L1551 (27.4768, -37.8905) -> (27.8455, -38.0872)
  line L1552 (27.1153, -37.6879) -> (27.4768, -37.8905)
  line L1553 (26.7611, -37.4792) -> (27.1153, -37.6879)
  line L1554 (26.4145, -37.2644) -> (26.7611, -37.4792)
  line L1555 (26.0759, -37.0434) -> (26.4145, -37.2644)
  line L1556 (28.603, -38.4628) -> (28.9916, -38.6418)
  line L1557 (28.9916, -38.6418) -> (29.3864, -38.815)
  line L1558 (29.3864, -38.815) -> (29.7874, -38.9823)
  line L1559 (29.7874, -38.9823) -> (30.1943, -39.1439)
  line L1560 (30.1943, -39.1439) -> (30.6071, -39.2996)
  line L1561 (30.6071, -39.2996) -> (30.8927, -39.0755)
  line L1562 (30.8927, -39.0755) -> (31.1767, -38.8493)
  line L1563 (31.1767, -38.8493) -> (31.459, -38.621)
  line L1564 (31.459, -38.621) -> (31.7397, -38.3907)
  line L1565 (31.7397, -38.3907) -> (32.0186, -38.1583)
  line L1566 (25.4241, -36.5817) -> (25.7456, -36.8158)
  line L1567 (18.2329, -34.6288) -> (18.1365, -34.8267)
  line L1568 (18.9686, -40.3088) -> (19.0107, -40.7043)
  line L1569 (18.9158, -39.9179) -> (18.9686, -40.3088)
  line L1570 (18.8516, -39.5322) -> (18.9158, -39.9179)
  line L1571 (18.7748, -39.1522) -> (18.8516, -39.5322)
  line L1572 (18.6839, -38.7788) -> (18.7748, -39.1522)
  line L1573 (18.576, -38.4134) -> (18.6839, -38.7788)
  line L1574 (19.0107, -40.7043) -> (19.0425, -41.1041)
  line L1575 (19.0425, -41.1041) -> (19.0647, -41.5079)
  line L1576 (19.0083, -44.0023) -> (18.969, -44.4283)
  line L1577 (19.0392, -43.579) -> (19.0083, -44.0023)
  line L1578 (19.0617, -43.1585) -> (19.0392, -43.579)
  line L1579 (19.0757, -42.7409) -> (19.0617, -43.1585)
  line L1580 (19.081, -42.3265) -> (19.0757, -42.7409)
  line L1581 (19.0774, -41.9154) -> (19.081, -42.3265)
  line L1582 (19.0647, -41.5079) -> (19.0774, -41.9154)
  line L1583 (18.969, -44.4283) -> (18.9216, -44.8569)
  line L1584 (18.866, -45.2878) -> (18.8024, -45.721)
  line L1585 (18.8024, -45.721) -> (18.7309, -46.1563)
  line L1586 (18.7309, -46.1563) -> (18.394, -46.2916)
  line L1587 (18.394, -46.2916) -> (18.0561, -46.4245)
  line L1588 (18.0561, -46.4245) -> (17.7172, -46.5548)
  line L1589 (17.7172, -46.5548) -> (17.3775, -46.6827)
  line L1590 (17.3775, -46.6827) -> (17.0368, -46.8081)
  line L1591 (18.9216, -44.8569) -> (18.866, -45.2878)
  line L1592 (18.3447, -34.4386) -> (18.2329, -34.6288)
  line L1593 (18.4826, -34.2517) -> (18.3447, -34.4386)
  line L1594 (18.6427, -34.0722) -> (18.4826, -34.2517)
  line L1595 (18.8473, -33.8913) -> (18.6427, -34.0722)
  line L1596 (19.1345, -33.6962) -> (18.8473, -33.8913)
  line L1597 (19.1827, -33.6688) -> (19.1345, -33.6962)
  line L1598 (19.2308, -33.6413) -> (19.1827, -33.6688)
  line L1599 (19.2789, -33.6138) -> (19.2308, -33.6413)
  line L1600 (19.327, -33.5862) -> (19.2789, -33.6138)
  line L1601 (19.375, -33.5585) -> (19.327, -33.5862)
  line L1602 (28.9985, -27.169) -> (29.0481, -27.381)
  line L1603 (29.0481, -27.381) -> (29.1106, -27.5952)
  line L1604 (29.1106, -27.5952) -> (29.1908, -27.806)
  line L1605 (29.1908, -27.806) -> (29.2872, -28.0147)
  line L1606 (29.395, -28.2257) -> (29.5186, -28.4343)
  line L1607 (29.5186, -28.4343) -> (29.6577, -28.6406)
  line L1608 (29.6577, -28.6406) -> (29.8119, -28.8444)
  line L1609 (29.8119, -28.8444) -> (29.9772, -29.0498)
  line L1610 (29.9772, -29.0498) -> (30.1555, -29.2545)
  line L1611 (29.6842, -24.908) -> (29.7198, -24.8655)
  line L1612 (29.7198, -24.8655) -> (29.7553, -24.823)
  line L1613 (29.7553, -24.823) -> (29.7908, -24.7804)
  line L1614 (29.7908, -24.7804) -> (29.8262, -24.7378)
  line L1615 (30.3482, -29.4569) -> (30.5939, -29.7434)
  circle A32 centre (0, 0) radius 45 construction
  circle A33 centre (0, 0) radius 45 construction
  line L1616 (29.8262, -24.7378) -> (29.8616, -24.6951)
  line L1617 (29.8616, -24.6951) -> (30.1036, -24.4461)
  line L1618 (30.1036, -24.4461) -> (30.3173, -24.2761)
  line L1619 (30.3173, -24.2761) -> (30.5219, -24.1496)
  line L1620 (30.5219, -24.1496) -> (30.7299, -24.0462)
  line L1621 (30.7299, -24.0462) -> (30.9366, -23.9692)
  line L1622 (30.9366, -23.9692) -> (31.1483, -23.9085)
  line L1623 (31.1483, -23.9085) -> (31.3597, -23.8696)
  line L1624 (31.3597, -23.8696) -> (31.575, -23.8461)
  line L1625 (31.575, -23.8461) -> (31.7918, -23.8401)
  line L1626 (31.7918, -23.8401) -> (32.0092, -23.8521)
  line L1627 (32.0092, -23.8521) -> (32.231, -23.8765)
  line L1628 (32.231, -23.8765) -> (32.4525, -23.9189)
  line L1629 (32.4525, -23.9189) -> (32.6748, -23.9775)
  line L1630 (32.6748, -23.9775) -> (32.9013, -24.0471)
  line L1631 (30.1555, -29.2545) -> (30.3482, -29.4569)
  line L1632 (32.9013, -24.0471) -> (33.1282, -24.1326)
  line L1633 (33.1282, -24.1326) -> (33.3555, -24.2337)
  line L1634 (33.3555, -24.2337) -> (33.583, -24.3502)
  line L1635 (33.583, -24.3502) -> (33.814, -24.4773)
  line L1636 (34.0465, -24.6174) -> (34.2792, -24.772)
  line L1637 (33.814, -24.4773) -> (34.0465, -24.6174)
  line L1638 (29.2872, -28.0147) -> (29.395, -28.2257)
  line L1639 (34.2792, -24.772) -> (34.6041, -24.9642)
  line L1640 (34.6041, -24.9642) -> (34.9452, -25.1339)
  line L1641 (35.2972, -25.2883) -> (35.6581, -25.4299)
  line L1642 (35.6581, -25.4299) -> (36.0268, -25.5601)
  line L1643 (36.0268, -25.5601) -> (36.4025, -25.68)
  line L1644 (34.9452, -25.1339) -> (35.2972, -25.2883)
  line L1645 (28.9667, -26.9545) -> (28.9985, -27.169)
  line L1646 (28.9541, -26.5234) -> (28.9525, -26.7384)
  line L1647 (28.9525, -26.7384) -> (28.9667, -26.9545)
  line L1648 (36.7847, -25.7901) -> (37.1729, -25.8909)
  line L1649 (39.6108, -26.3174) -> (40.0331, -26.3604)
  line L1650 (39.1928, -26.2665) -> (39.6108, -26.3174)
  line L1651 (38.7791, -26.2078) -> (39.1928, -26.2665)
  line L1652 (38.3701, -26.1411) -> (38.7791, -26.2078)
  line L1653 (37.9659, -26.0661) -> (38.3701, -26.1411)
  line L1654 (37.5667, -25.9828) -> (37.9659, -26.0661)
  line L1655 (37.1729, -25.8909) -> (37.5667, -25.9828)
  line L1656 (40.0331, -26.3604) -> (40.4594, -26.3957)
  line L1657 (40.4594, -26.3957) -> (40.8897, -26.4234)
  line L1658 (40.8897, -26.4234) -> (41.3237, -26.4435)
  line L1659 (41.3237, -26.4435) -> (41.7614, -26.4561)
  line L1660 (41.7614, -26.4561) -> (42.2025, -26.4613)
  line L1661 (42.2025, -26.4613) -> (42.3943, -26.153)
  line L1662 (42.3943, -26.153) -> (42.5838, -25.8433)
  line L1663 (42.5838, -25.8433) -> (42.771, -25.5322)
  line L1664 (42.771, -25.5322) -> (42.9559, -25.2198)
  line L1665 (42.9559, -25.2198) -> (43.1386, -24.9061)
  line L1666 (36.4025, -25.68) -> (36.7847, -25.7901)
  line L1667 (28.9771, -26.3044) -> (28.9541, -26.5234)
  line L1668 (31.6111, -31.3902) -> (31.7858, -31.7475)
  line L1669 (31.4278, -31.041) -> (31.6111, -31.3902)
  line L1670 (31.2355, -30.7005) -> (31.4278, -31.041)
  line L1671 (31.0334, -30.3697) -> (31.2355, -30.7005)
  line L1672 (30.8202, -30.0499) -> (31.0334, -30.3697)
  line L1673 (30.5939, -29.7434) -> (30.8202, -30.0499)
  line L1674 (31.7858, -31.7475) -> (31.9525, -32.1123)
  line L1675 (31.9525, -32.1123) -> (32.1115, -32.4841)
  line L1676 (32.9116, -34.8475) -> (33.0204, -35.2612)
  line L1677 (32.7959, -34.4391) -> (32.9116, -34.8475)
  line L1678 (32.6732, -34.0362) -> (32.7959, -34.4391)
  line L1679 (32.5436, -33.639) -> (32.6732, -34.0362)
  line L1680 (32.4068, -33.2478) -> (32.5436, -33.639)
  line L1681 (32.2628, -32.8628) -> (32.4068, -33.2478)
  line L1682 (32.1115, -32.4841) -> (32.2628, -32.8628)
  line L1683 (33.0204, -35.2612) -> (33.1224, -35.6801)
  line L1684 (33.2176, -36.1041) -> (33.306, -36.5329)
  line L1685 (33.306, -36.5329) -> (33.3877, -36.9664)
  line L1686 (33.3877, -36.9664) -> (33.1173, -37.2088)
  line L1687 (33.1173, -37.2088) -> (32.8453, -37.4492)
  line L1688 (32.8453, -37.4492) -> (32.5715, -37.6876)
  line L1689 (32.5715, -37.6876) -> (32.2959, -37.924)
  line L1690 (32.2959, -37.924) -> (32.0186, -38.1583)
  line L1691 (33.1224, -35.6801) -> (33.2176, -36.1041)
  line L1692 (29.0171, -26.0875) -> (28.9771, -26.3044)
  line L1693 (29.0828, -25.8646) -> (29.0171, -26.0875)
  line L1694 (29.1718, -25.6412) -> (29.0828, -25.8646)
  line L1695 (29.3021, -25.4012) -> (29.1718, -25.6412)
  line L1696 (29.5054, -25.1196) -> (29.3021, -25.4012)
  line L1697 (29.5412, -25.0774) -> (29.5054, -25.1196)
  line L1698 (29.5771, -25.0351) -> (29.5412, -25.0774)
  line L1699 (29.6129, -24.9928) -> (29.5771, -25.0351)
  line L1700 (29.6486, -24.9504) -> (29.6129, -24.9928)
  line L1701 (29.6842, -24.908) -> (29.6486, -24.9504)
  line L1702 (36.5421, -15.6124) -> (36.6611, -15.7947)
  line L1703 (36.6611, -15.7947) -> (36.7931, -15.9746)
  line L1704 (36.7931, -15.9746) -> (36.9406, -16.1452)
  line L1705 (36.9406, -16.1452) -> (37.1025, -16.3084)
  line L1706 (37.2761, -16.4698) -> (37.4636, -16.6236)
  line L1707 (37.4636, -16.6236) -> (37.6648, -16.7698)
  line L1708 (37.6648, -16.7698) -> (37.8794, -16.9086)
  line L1709 (37.8794, -16.9086) -> (38.105, -17.0451)
  line L1710 (38.105, -17.0451) -> (38.3425, -17.1764)
  line L1711 (36.4131, -13.2533) -> (36.432, -13.2012)
  line L1712 (36.432, -13.2012) -> (36.4508, -13.1491)
  line L1713 (36.4508, -13.1491) -> (36.4696, -13.0969)
  line L1714 (36.4696, -13.0969) -> (36.4883, -13.0448)
  line L1715 (38.5928, -17.3007) -> (38.9217, -17.4859)
  circle A34 centre (0, 0) radius 45 construction
  circle A35 centre (0, 0) radius 45 construction
  line L1716 (36.4883, -13.0448) -> (36.5069, -12.9926)
  line L1717 (36.5069, -12.9926) -> (36.6492, -12.6758)
  line L1718 (36.6492, -12.6758) -> (36.7919, -12.4429)
  line L1719 (36.7919, -12.4429) -> (36.9408, -12.2541)
  line L1720 (36.9408, -12.2541) -> (37.1009, -12.0858)
  line L1721 (37.1009, -12.0858) -> (37.2688, -11.9427)
  line L1722 (37.2688, -11.9427) -> (37.447, -11.8133)
  line L1723 (37.447, -11.8133) -> (37.6324, -11.7044)
  line L1724 (37.6324, -11.7044) -> (37.8267, -11.6087)
  line L1725 (37.8267, -11.6087) -> (38.0283, -11.529)
  line L1726 (38.0283, -11.529) -> (38.2367, -11.4659)
  line L1727 (38.2367, -11.4659) -> (38.4534, -11.4129)
  line L1728 (38.4534, -11.4129) -> (38.6761, -11.377)
  line L1729 (38.6761, -11.377) -> (38.905, -11.3561)
  line L1730 (38.905, -11.3561) -> (39.1417, -11.344)
  line L1731 (38.3425, -17.1764) -> (38.5928, -17.3007)
  line L1732 (39.1417, -11.344) -> (39.3842, -11.3467)
  line L1733 (39.3842, -11.3467) -> (39.6323, -11.364)
  line L1734 (39.6323, -11.364) -> (39.886, -11.3956)
  line L1735 (39.886, -11.3956) -> (40.1465, -11.4361)
  line L1736 (40.4129, -11.4882) -> (40.6845, -11.5538)
  line L1737 (40.1465, -11.4361) -> (40.4129, -11.4882)
  line L1738 (37.1025, -16.3084) -> (37.2761, -16.4698)
  line L1739 (40.6845, -11.5538) -> (41.0555, -11.6234)
  line L1740 (41.0555, -11.6234) -> (41.4341, -11.6662)
  line L1741 (41.8176, -11.6908) -> (42.2052, -11.7005)
  line L1742 (42.2052, -11.7005) -> (42.5962, -11.6968)
  line L1743 (42.5962, -11.6968) -> (42.9903, -11.6809)
  line L1744 (41.4341, -11.6662) -> (41.8176, -11.6908)
  line L1745 (36.4388, -15.4218) -> (36.5421, -15.6124)
  line L1746 (36.2795, -15.0209) -> (36.3516, -15.2235)
  line L1747 (36.3516, -15.2235) -> (36.4388, -15.4218)
  line L1748 (43.387, -11.6536) -> (43.7863, -11.6156)
  line L1749 (46.223, -11.1825) -> (46.6346, -11.0786)
  line L1750 (45.8128, -11.2778) -> (46.223, -11.1825)
  line L1751 (45.4041, -11.3641) -> (45.8128, -11.2778)
  line L1752 (44.9969, -11.4412) -> (45.4041, -11.3641)
  line L1753 (44.5914, -11.509) -> (44.9969, -11.4412)
  line L1754 (44.1878, -11.5673) -> (44.5914, -11.509)
  line L1755 (43.7863, -11.6156) -> (44.1878, -11.5673)
  line L1756 (46.6346, -11.0786) -> (47.0473, -10.9659)
  line L1757 (47.0473, -10.9659) -> (47.4611, -10.8448)
  line L1758 (47.4611, -10.8448) -> (47.8758, -10.7152)
  line L1759 (47.8758, -10.7152) -> (48.2914, -10.5774)
  line L1760 (48.2914, -10.5774) -> (48.7077, -10.4313)
  line L1761 (48.7077, -10.4313) -> (48.7824, -10.0761)
  line L1762 (48.7824, -10.0761) -> (48.8546, -9.7203)
  line L1763 (48.8546, -9.7203) -> (48.9241, -9.3639)
  line L1764 (48.9241, -9.3639) -> (48.9911, -9.0071)
  line L1765 (48.9911, -9.0071) -> (49.0554, -8.6498)
  line L1766 (42.9903, -11.6809) -> (43.387, -11.6536)
  line L1767 (36.2262, -14.8073) -> (36.2795, -15.0209)
  line L1768 (40.4408, -18.6855) -> (40.7272, -18.9615)
  line L1769 (40.1491, -18.4201) -> (40.4408, -18.6855)
  line L1770 (39.852, -18.1659) -> (40.1491, -18.4201)
  line L1771 (39.5489, -17.9241) -> (39.852, -18.1659)
  line L1772 (39.2392, -17.6965) -> (39.5489, -17.9241)
  line L1773 (38.9217, -17.4859) -> (39.2392, -17.6965)
  line L1774 (40.7272, -18.9615) -> (41.0086, -19.2472)
  line L1775 (41.0086, -19.2472) -> (41.2851, -19.5423)
  line L1776 (42.8453, -21.4895) -> (43.0891, -21.841)
  line L1777 (42.5969, -21.1453) -> (42.8453, -21.4895)
  line L1778 (42.3439, -20.8086) -> (42.5969, -21.1453)
  line L1779 (42.0862, -20.4798) -> (42.3439, -20.8086)
  line L1780 (41.8239, -20.1589) -> (42.0862, -20.4798)
  line L1781 (41.5569, -19.8464) -> (41.8239, -20.1589)
  line L1782 (41.2851, -19.5423) -> (41.5569, -19.8464)
  line L1783 (43.0891, -21.841) -> (43.3282, -22.1998)
  line L1784 (43.5626, -22.5656) -> (43.7924, -22.9383)
  line L1785 (43.7924, -22.9383) -> (44.0174, -23.3178)
  line L1786 (44.0174, -23.3178) -> (43.8463, -23.638)
  line L1787 (43.8463, -23.638) -> (43.6728, -23.957)
  line L1788 (43.6728, -23.957) -> (43.4971, -24.2746)
  line L1789 (43.4971, -24.2746) -> (43.319, -24.591)
  line L1790 (43.319, -24.591) -> (43.1386, -24.9061)
  line L1791 (43.3282, -22.1998) -> (43.5626, -22.5656)